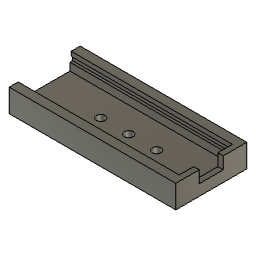
ESP-PROG Holder v1 (Autodesk Fusion 360 design; units mm, degrees)
Autodesk Fusion 360 part; units mm, degrees
sketch "Main Body" plane through (0, 0, 0) normal (1, 0, 0) x (0, 1, 0)
  line L0 (0, 0) -> (16.2, 0)
  line L1 (16.2, 0) -> (16.2, 10.5)
  line L2 (16.2, 10.5) -> (12.1, 10.5)
  line L3 (12.1, 10.5) -> (12.1, 8.5)
  line L4 (12.1, 8.5) -> (12.7, 8.5)
  line L5 (12.7, 8.5) -> (12.7, 6.5)
  line L6 (12.7, 6.5) -> (11.5, 6.5)
  line L7 (11.5, 6.5) -> (11.5, 3)
  line L8 (11.5, 3) -> (0, 3)
  line L9 (0, 35) -> (0, -40) construction
  line L10 (-12.1, 10.5) -> (-12.1, 8.5)
  line L11 (-11.5, 6.5) -> (-11.5, 3)
  line L12 (-12.1, 8.5) -> (-12.7, 8.5)
  line L13 (-12.7, 6.5) -> (-11.5, 6.5)
  line L14 (-12.7, 8.5) -> (-12.7, 6.5)
  line L15 (-16.2, 10.5) -> (-12.1, 10.5)
  line L16 (-16.2, 0) -> (-16.2, 10.5)
  line L17 (0, 0) -> (-16.2, 0)
  line L18 (-11.5, 3) -> (0, 3)
  dimension "d1" = 16.2
  dimension "d4" = 4.1
  dimension "d5" = 0.6
  dimension "d6" = 2
  dimension "d9" = 4.7
  dimension "d10" = 6.5
  dimension "d11" = 2
  dimension "d16" = 3
  constraint horizontal L0
  constraint perpendicular L0 L1
  constraint perpendicular L1 L2
  constraint perpendicular L0 L3
  constraint perpendicular L3 L4
  constraint perpendicular L4 L5
  constraint perpendicular L5 L6
  constraint perpendicular L6 L7
  constraint perpendicular L7 L8
  constraint coincident L0.start L17.start
  constraint vertical L9
  constraint coincident L8.end L9
  constraint symmetric L0.start L9 L17.start
  constraint symmetric L0.end L9 L16.start
  constraint symmetric L1.end L9 L15.start
  constraint symmetric L2.end L9 L10.start
  constraint symmetric L3.end L9 L10.end
  constraint symmetric L4.end L9 L12.end
  constraint symmetric L5.end L9 L13.start
  constraint symmetric L6.end L9 L11.start
  constraint symmetric L7.end L9 L11.end
  constraint symmetric L8.end L9 L18.end
  measures "d1" distance of L0.start L0.end
  measures "d4" distance of L1.end L2.end
  measures "d5" distance of L3.end L4.end
  measures "d6" distance of L4.end L5.end
  measures "d9" distance of L1 L7
  measures "d10" distance of L0 L6
  measures "d11" distance of L2 L4
  measures "d16" distance of L0 L8
extrude "Extrude1" add sketch "Main Body" along normal blind 76
sketch "USB Endstop" plane through (76, 0, 0) normal (1, 0, 0) x (0, 1, 0)
  line L0 (-16.2, 0) -> (16.2, 0)
  line L1 (16.2, 0) -> (16.2, 10.5)
  line L2 (16.2, 10.5) -> (12.1, 10.5)
  line L3 (12.1, 10.5) -> (12.1, 8.5)
  line L4 (12.1, 8.5) -> (12.7, 8.5)
  line L5 (12.7, 8.5) -> (12.7, 6.5)
  line L6 (12.7, 6.5) -> (11.5, 6.5)
  line L7 (11.5, 6.5) -> (11.5, 3)
  line L8 (11.5, 3) -> (-11.5, 3)
  line L9 (-11.5, 3) -> (-11.5, 6.5)
  line L10 (-11.5, 6.5) -> (-12.7, 6.5)
  line L11 (-12.7, 6.5) -> (-12.7, 8.5)
  line L12 (-12.7, 8.5) -> (-12.1, 8.5)
  line L13 (-12.1, 8.5) -> (-12.1, 10.5)
  line L14 (-12.1, 10.5) -> (-16.2, 10.5)
  line L15 (-16.2, 10.5) -> (-16.2, 0)
  line L16 (0, 5) -> (5.5, 5)
  line L17 (5.5, 5) -> (5.5, 10.5)
  line L18 (5.5, 10.5) -> (12.1, 10.5)
  line L19 (0, 12) -> (0, -4) construction
  line L20 (-5.5, 5) -> (-5.5, 10.5)
  line L21 (-5.5, 10.5) -> (-12.1, 10.5)
  line L22 (0, 5) -> (-5.5, 5)
  dimension "d14" = 5.5
  dimension "d15" = 5
  constraint horizontal L16
  constraint perpendicular L16 L17
  constraint coincident L2.end L3.start
  constraint horizontal L18
  constraint perpendicular L0 L19
  constraint coincident L16.start L19
  constraint symmetric L16.start L19 L22.start
  constraint symmetric L16.end L19 L20.start
  constraint symmetric L17.end L19 L20.end
  constraint symmetric L2.end L19 L13.end
  measures "d14" distance of L16.start L16.end
  measures "d15" distance of L0 L16
extrude "Extrude2" add sketch "USB Endstop" against normal blind 2.5 contours L3 L4 L5 L6 L7 L8 L9 L10 L11 L12 L13 L16 L17 L18 L20 L21 L22
sketch "DIN Holes" plane through (0, 0, 0) normal (0, 0, -1) x (1, 0, 0)
  line L0 (0, 16.2) -> (0, -16.2)
  line L1 (0, -16.2) -> (76, -16.2)
  line L2 (76, -16.2) -> (76, 16.2)
  line L3 (76, 16.2) -> (0, 16.2)
  line L4 (0, 16) -> (76, -16.2) construction
  line L5 (76.7439, 16.2) -> (0, -16.2) construction
  circle A0 centre (38.372, 0) radius 2
  circle A1 centre (25.622, 0) radius 2
  circle A2 centre (51.122, 0) radius 2
  dimension "d20" = 4
  dimension "d23" = 12.75
  dimension "d24" = 0
  constraint coincident L0 L4.start
  constraint coincident L1.end L2.start
  constraint coincident L3 L5.start
  constraint coincident L0.end L1.start
  constraint midpoint L5 A0.centre
  measures "d20" diameter of A0
extrude "Extrude3" cut sketch "DIN Holes" against normal up to surface (3 mm away) contours A0 | A1 | A2
